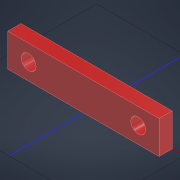
# Autodesk Inventor part: BMP280_Cableclamp
Saved by Autodesk Inventor 2022 (Build 260153000, 153)
## iProperties
Created: 2022-02-02
Part Number: BMP280_Cableclamp
Material: Generisch
Document SubType Name: Modeling
Designer: sleib
Density: 1 g/cm^3
Appearance: Rot
Author: sleib
Autodesk Inventor part; units mm, degrees
ref_plane "YZ Plane" through (0, 0, 0) normal (1, 0, 0) x (0, 1, 0)
ref_plane "XZ Plane" through (0, 0, 0) normal (0, 1, 0) x (-1, 0, 0)
ref_plane "XY Plane" through (0, 0, 0) normal (0, 0, 1) x (1, 0, 0)
sketch "Skizze1" plane through (0, 0, 0) normal (0, 0, 1) x (1, 0, 0)
  line L0 (-17.25, -3.75) -> (17.25, -3.75)
  line L1 (17.25, -3.75) -> (17.25, 3.75)
  line L2 (17.25, 3.75) -> (-17.25, 3.75)
  line L3 (-17.25, 3.75) -> (-17.25, -3.75)
  line L4 (-17.25, -3.75) -> (17.25, 3.75) construction
  line L5 (17.25, -3.75) -> (-17.25, 3.75) construction
  circle A0 centre (-12.5, 0) radius 1.7
  circle A1 centre (12.5, 0) radius 1.7
  line L6 (-17.25, 0) -> (17.25, 0) construction
  line L7 (0, -5.25) -> (0, 5.25) construction
  point P0 (0, 0)
  dimension "d0" = 7.5
  dimension "d1" = 34.5
  dimension "d2" = 3.4
  dimension "d3" = 25
  constraints: 14 end point, 4 midpoint, 2 centre point, 2 parallel, 2 point on line, 1 equal radius, 1 horizontal, 1 perpendicular, 1 symmetric about line
  measures "d0" distance of L2.end L0.start
  measures "d1" distance of L1.end L2.end
  measures "d2" diameter of A0
  measures "d3" distance of A1.centre A0.centre
extrude "Extrusion1" add sketch "Skizze1" along normal blind 3
